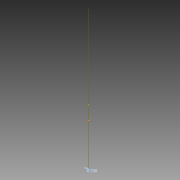
# Autodesk Inventor part: OCT_Probe
Saved by Autodesk Inventor 2011 SP2 (Build 150309200, 309)
## iProperties
Created: 2012-03-27
Part Number: OCT_Probe
Document SubType Name: Modeling
Designer: sungwook
Density: 1 g/cm^3
Author: sungwook
Autodesk Inventor part; units mm, degrees
ref_plane "YZ Plane" through (0, 0, 0) normal (1, 0, 0) x (0, 1, 0)
ref_plane "XZ Plane" through (0, 0, 0) normal (0, 1, 0) x (-1, 0, 0)
ref_plane "XY Plane" through (0, 0, 0) normal (0, 0, 1) x (1, 0, 0)
sketch "Sketch1" plane through (0, 0, 0) normal (0, 0, 1) x (1, 0, 0)
  circle A0 centre (0, 0) radius 0.254
  dimension "d0" = 0.508
  constraints: 1 centre point, 1 coincident
  measures "d0" diameter of A0
extrude "Extrusion1" add sketch "Sketch1" along normal blind 60
ref_plane "Work Plane1" through (0, 0, 80) normal (0, 0, 1) x (1, 0, 0)
sketch "Sketch2" plane through (0, 0, 80) normal (0, 0, 1) x (1, 0, 0)
  circle A0 centre (0, 0) radius 0.254
  dimension "d4" = 0.508
  constraints: 1 centre point, 1 coincident
  measures "d4" diameter of A0
sketch "Sketch3" plane through (0, 0, 0) normal (0, 1, 0) x (-1, 0, 0)
  line L0 (0, -16) -> (0, 96) projected
  line L1 (-0.254, 60) -> (0.254, 60) projected
  line L2 (-0.506, 80) -> (0.9159, 80) projected
  spline S0 degree 4 poles (0, 60) (0, 61.9564) (-0.4751, 64.4982) (1.601, 74.5143) (0, 77.6037) (0, 80) knots 0 0 0 0 0 0.488556 1 1 1 1 1
  line L3 (0, 60) -> (0, 58.4828)
  line L4 (0, 80) -> (0, 96.834)
  point P0 (0, 0)
  point P1 (0, 64.3838)
  point P2 (0.5789, 74.0552)
  constraints: 5 point on line, 4 end point, 2 vertical, 1 midpoint, 4 other
sketch "Sketch4" plane through (0, 0, 60) normal (0, 0, 1) x (1, 0, 0)
  circle A0 centre (0, 0) radius 0.254 projected
sweep "Sweep1" add profiles "Sketch2" path "Sketch3" path curves L4 S0 L3
sketch "Sketch5" plane through (0, 0, 96.834) normal (0, 0, 1) x (1, 0, 0)
  circle A0 centre (0, 0) radius 0.254 projected
extrude "Extrusion2" add sketch "Sketch5" along normal blind 100
body "Solid1"
